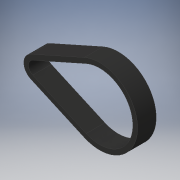
# Autodesk Inventor part: Belt
Saved by Autodesk Inventor 2019.4 (Build 234330000, 330)
## iProperties
Created: 2019-03-02
Part Number: Belt
Material: Rubber, Silicone
Document SubType Name: Modeling
Designer: Petar
Density: 1.25 g/cm^3
Appearance: Rubber - Black
Mass: 9.72075 g
Surface Area: 81.0652 cm^2
Volume: 7.7766 cm^3
Author: Petar
Autodesk Inventor part; units mm, degrees
ref_plane "YZ Plane" through (0, 0, 0) normal (1, 0, 0) x (0, 1, 0)
ref_plane "XZ Plane" through (0, 0, 0) normal (0, 1, 0) x (-1, 0, 0)
ref_plane "XY Plane" through (0, 0, 0) normal (0, 0, 1) x (1, 0, 0)
sketch "Sketch1" plane through (0, 0, 0) normal (0, 0, 1) x (1, 0, 0)
  circle A0 centre (0, 0) radius 7.26 construction
  line L0 (0, 0) -> (51.5, 0) construction
  arc A1 (-2.3048, 5.1684) -> (-2.3048, -5.1684) centre (0, 0) ccw
  arc A2 (9.469, 0) -> (4.6289, 8.2604) centre (0, 0) ccw construction
  circle A3 centre (51.5, 0) radius 28.265 construction
  arc A4 (40.6525, -24.3249) -> (40.6525, 24.3249) centre (51.5, 0) ccw
  arc A5 (21.056, 0) -> (27.1842, -18.3188) centre (51.5, 0) ccw construction
  line L1 (-3.8565, 8.6481) -> (39.1007, 27.8046)
  line L2 (-3.8565, -8.6481) -> (39.1007, -27.8046)
  line L3 (-2.3048, 5.1684) -> (40.6525, 24.3249)
  line L4 (-2.3048, -5.1684) -> (40.6525, -24.3249)
  arc A6 (24.866, 0) -> (40.6525, -24.3249) centre (51.5, 0) ccw construction
  arc A7 (40.6525, 24.3249) -> (24.866, 0) centre (51.5, 0) ccw construction
  arc A8 (5.659, 0) -> (-2.3048, 5.1684) centre (0, 0) ccw construction
  arc A9 (-2.3048, -5.1684) -> (5.659, 0) centre (0, 0) ccw construction
  arc A10 (4.6289, -8.2604) -> (9.469, 0) centre (0, 0) ccw construction
  arc A11 (4.6289, 8.2604) -> (-3.8565, 8.6481) centre (0, 0) ccw construction
  arc A12 (27.1842, 18.3188) -> (21.056, 0) centre (51.5, 0) ccw construction
  arc A13 (27.1842, -18.3188) -> (39.1007, -27.8046) centre (51.5, 0) ccw construction
  arc A14 (-3.8565, 8.6481) -> (-3.8565, -8.6481) centre (0, 0) ccw
  arc A15 (-3.8565, -8.6481) -> (4.6289, -8.2604) centre (0, 0) ccw construction
  arc A16 (39.1007, 27.8046) -> (27.1842, 18.3188) centre (51.5, 0) ccw construction
  arc A17 (39.1007, -27.8046) -> (39.1007, 27.8046) centre (51.5, 0) ccw
  dimension "d0" = 14.52
  dimension "d1" = 51.5
  dimension "d4" = 56.53
  dimension "d10" = 3.81
  dimension "d12" = 3.81
  dimension "d13" = 1.601
  dimension "d14" = 1.631
  constraints: 34 point on circle, 18 centre point, 12 tangent, 10 end point, 8 point on line, 6 coincident, 4 symmetric about line, 1 horizontal
  measures "d0" diameter of A0
  measures "d1" distance of L0.start L0.end
  measures "d4" diameter of A3
  measures "d10" radial gap between concentric circles of A17 A4
  measures "d12" radial gap between concentric circles of A14 A1
  measures "d13" radial gap between concentric circles of A1 A0
  measures "d14" radial gap between concentric circles of A4 A3
extrude "Extrusion1" add sketch "Sketch1" along normal blind 15
body "Solid1"
